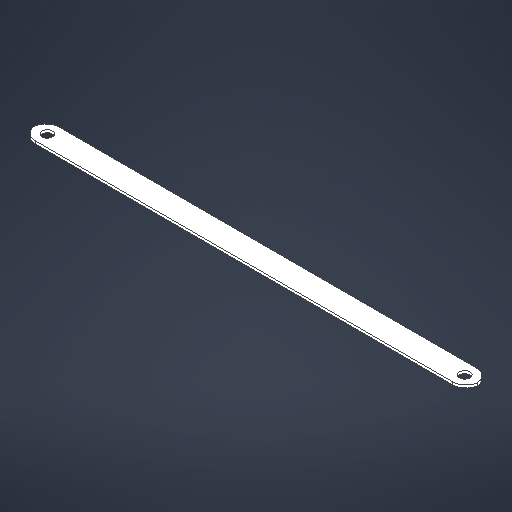
# Autodesk Inventor part: Pieza40
Saved by Autodesk Inventor 2026.2 (Build 302298000, 298)
## iProperties
Created: 2026-01-02
Part Number: Pieza40
Material: Genérico
Document SubType Name: Modeling
Designer: vicho
Density: 1 g/cm^3
Appearance: Valor por defecto
Author: vicho
Autodesk Inventor part; units mm, degrees
ref_plane "YZ Plane" through (0, 0, 0) normal (1, 0, 0) x (0, 1, 0)
ref_plane "XZ Plane" through (0, 0, 0) normal (0, 1, 0) x (-1, 0, 0)
ref_plane "XY Plane" through (0, 0, 0) normal (0, 0, 1) x (1, 0, 0)
sketch "Boceto1" plane through (0, 0, 0) normal (0, 1, 0) x (-1, 0, 0)
  line L0 (385.7227, 0) -> (-335.8409, 0) construction
  line L1 (0, 516.0097) -> (0, -537.3218) construction
  line L2 (-157.5, -9) -> (157.5, -9)
  line L3 (167.5, 1) -> (167.5, -1)
  line L4 (157.5, 9) -> (-157.5, 9)
  line L5 (-167.5, -1) -> (-167.5, 1)
  line L6 (-167.5, -9) -> (167.5, 9) construction
  line L7 (167.5, -9) -> (-167.5, 9) construction
  arc A0 (167.5, -1) -> (157.5, 9) centre (157.5, -1) ccw
  arc A1 (157.5, -9) -> (167.5, 1) centre (157.5, 1) ccw
  arc A2 (-167.5, 1) -> (-157.5, -9) centre (-157.5, 1) ccw
  arc A3 (-157.5, 9) -> (-167.5, -1) centre (-157.5, -1) ccw
  line L8 (157.5, 9) -> (157.5, -15.4925) construction
  circle A4 centre (157.5, 0) radius 4
  line L9 (-157.5, -9) -> (-157.5, 29.1929) construction
  circle A5 centre (-157.5, 0) radius 4
  point P0 (0, 0)
  point P1 (167.4499, 0)
  point P2 (-167.4499, 0)
  dimension "d0" = 18
  dimension "d1" = 335
  dimension "d2" = 10
  dimension "d3" = 8
  dimension "d4" = 8
  constraints: 20 end point, 14 point on line, 8 point on circle, 8 tangent, 6 centre point, 3 equal radius, 3 vertical, 2 horizontal, 2 midpoint, 2 parallel, 1 perpendicular
  measures "d0" distance between parallel lines of L2 L4
  measures "d1" distance between parallel lines of L3 L5
  measures "d2" radius of A0
  measures "d3" diameter of A4
  measures "d4" diameter of A5
extrude "Extrusión1" add sketch "Boceto1" along normal blind 2 contours A2 A3 L4 A0 A1 L2
